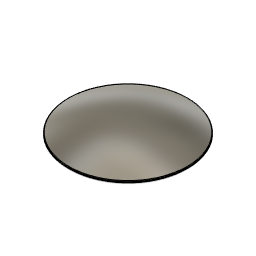
Convex_Topper_v0.9 (Autodesk Fusion 360 design; units mm, degrees)
Autodesk Fusion 360 part; units mm, degrees
note: some values were not read from the file. Set by a fixed rule: which sketch regions a step uses; which face or edge a step refers to.
sketch "Diameter" plane through (0, 0, 0) normal (0, 1, 0) x (1, 0, 0)
  circle A0 centre (0, 0) radius 50
  dimension "d3" = 100
  constraint coincident A0.centre origin
  measures "d3" diameter of A0
extrude "Extrude1" add sketch "Diameter" along normal blind 2
sketch "Dome" plane through (0, 0, 0) normal (0, 0, 1) x (1, 0, 0)
  line L0 (50, 2) -> (-50, 2)
  circle A0 centre (0, -132.3889) radius 143.3889
  line L1 (0, 0) -> (0, -132.3889) construction
  line L2 (0, 0) -> (0, 11)
  dimension "d6" = 11
  constraint coincident L0.end A0
  constraint coincident L1.start L2.start
  constraint coincident A0.centre L1.end
  constraint vertical L1
  constraint coincident A0 L2.end
  constraint perpendicular L0 L2
  measures "d6" distance of L1.start L2.end
revolve "Revolve1" add sketch "Dome" angle 360 about axis through (0, 0, 0) along (0, 1, 0) contours L0 A0 L2 picked at (5.6615, 7.6635)
chamfer "Chamfer1" distance 1 angle 45 1 edges at (-46.6164, 0, 18.0808)
chamfer "Chamfer1" distance 0.4 angle 45 1 edges at (-46.6164, 2, 18.0808)
sketch "Cutout for Threads" plane through (0, 0, 0) normal (0, -1, 0) x (1, 0, 0)
  circle A0 centre (0, 0) radius 49
  circle A1 centre (0, 0) radius 14
  dimension "d10" = 28
  constraint coincident A0.centre A1.centre
  measures "d10" diameter of A1
extrude "Extrude2" cut sketch "Cutout for Threads" against normal blind 6 contours A1
sketch "Cutout for Collet" plane through (0, 6, 0) normal (0, -1, 0) x (1, 0, 0)
  circle A0 centre (0, 0) radius 9
  circle A1 centre (0, 0) radius 14
  dimension "d13" = 18
  constraint coincident A0.centre A1.centre
  measures "d13" diameter of A0
extrude "Extrude3" cut sketch "Cutout for Collet" against normal blind 3 contours A0
sketch "Chamfer for Collet" plane through (0, 0, 0) normal (0, 0, 1) x (1, 0, 0)
  line L0 (9, 6) -> (-9, 6)
  line L1 (9, 6) -> (7.6706, 9)
  line L2 (9, 9) -> (9, 6)
  line L3 (0, 6) -> (0, 8)
  line L4 (9, 9) -> (-9, 9)
  constraint coincident L0.start L1.start
  constraint midpoint L0 L3.start
  constraint perpendicular L0 L3
revolve "Revolve2" add sketch "Chamfer for Collet" angle 360 about axis through (0, 6, 0) along (0, 1, 0)
sketch "Unsupported Hole" plane through (0, 6, 0) normal (0, -1, 0) x (1, 0, 0)
  circle A0 centre (0, 0) radius 9
  line L0 (-13.2288, 9) -> (13.2288, 9)
  line L1 (9, 13.2288) -> (9, -13.2288)
  line L2 (13.2288, -9) -> (-13.2288, -9)
  line L3 (-9, -13.2288) -> (-9, 13.2288)
  circle A1 centre (0, 0) radius 16
  dimension "d23" = 32
  constraint horizontal L0
  constraint perpendicular L0 L1
  constraint horizontal L2
  constraint perpendicular L2 L3
  constraint tangent A0 L3
  constraint tangent A0 L2
  constraint tangent A0 L0
  constraint tangent A0 L1
  constraint coincident L3.start A1
  constraint coincident L2.end A1
  constraint coincident L0.start A1
  constraint coincident L3.end A1
  constraint coincident L1.start A1
  constraint coincident L0.end A1
  constraint coincident L2.start A1
  constraint coincident L1.end A1
  measures "d23" diameter of A1
extrude "Extrude4" cut sketch "Unsupported Hole" against normal blind 0.4 contours A0 | A0 L1 L2 | A0 L0 L1 | A0 L0 L3 | A0 L2 L3
extrude "Extrude5" cut sketch "Unsupported Hole" against normal blind 0.2 contours L0 L1 L2 A1 | L0 L2 L3 A1
chamfer "Chamfer2" distance 0.4 angle 45 1 edges at (-8.2257, 6.4, -3.1904)
thread "Thread1" "ISO Metric profile 28.0 M28x2 6H" major diameter 28.2565 minor diameter 26.0224 pitch 2 angle 60 modelled right hand crest width 0.5434 on face at (0, 2, 14) crest through (13.0112, 0.5, 0)
extrude "Extrude6" add 2 faces at (-13.1114, 6, 7.3172) (13.1114, 6, 7.3172) along direction (0, 1, 0) blind 0.4
equation "Diameter = 100 mm" comment "Minimum 40mm"
equation "Peak_Height = 11 mm" comment "Minimum 11mm"
equation "d3 = Diameter"
equation "d6 = Peak_Height"
named bodies: "Convex Topper"
